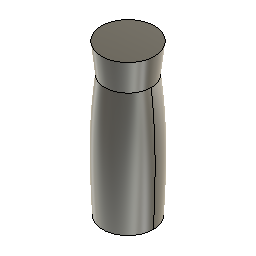
bicycle and bottle_final (Autodesk Fusion 360 archive; units mm, degrees)
design "Bottle"
Autodesk Fusion 360 part; units mm, degrees
sketch "Sketch2" plane through (0, 0, 0) normal (0, 1, 0) x (1, 0, 0)
  line L0 (0, 0) -> (0, -210)
  line L1 (0, -210) -> (36.8, -210)
  line L2 (36.8, -210) -> (32.35, -170)
  line L3 (35.4, 0) -> (0, 0)
  line L4 (32.35, -170) -> (0, -170) construction
  spline S0 degree 5 poles (32.35, -170) (32.7061, -167.196) (33.3914, -161.5338) (34.3388, -152.8777) (35.4383, -141.0057) (36.5224, -125.5792) (37.294, -109.5216) (37.7338, -92.7939) (37.8425, -75.3974) (37.643, -57.3785) (37.1635, -38.7939) (36.5763, -23.5151) (36.029, -11.8401) (35.6175, -3.9624) (35.4, 0) knots 0 0 0 0 0 0 0.1 0.2 0.3 0.4 0.5 0.6 0.7 0.8 0.9 1 1 1 1 1 1
  point P0 (37.5, -100)
  dimension "d13" = 210
  dimension "d14" = 35.4
  dimension "d15" = 36.8
  dimension "d16" = 32.35
  dimension "d18" = 170
  dimension "d20" = 37.5
  dimension "d21" = 100
  constraint coincident L0.start L3.end
  constraint vertical L0
  constraint perpendicular L0 L1
  constraint perpendicular L0 L3
  constraint coincident L0 L4.end
  constraint perpendicular L0 L4
  measures "d13" distance of L0.start L0.end
  measures "d14" distance of L3.start L0.start
  measures "d15" distance of L0.end L1.end
  measures "d16" distance of L0 L2.end
  measures "d18" distance of L3 L4
  measures "d20" distance of L0 P0
  measures "d21" distance of L3 P0
revolve "Revolve1" add sketch "Sketch2" angle 360 about axis through (0, 0, 0) along (0, 0, 1)
equation "overallHeight = 210 mm"
equation "bottomDiameter = ( 70.8 / 2 ) * 1 mm"
equation "bottleCapTop = ( 73.6 / 2 ) * 1 mm"
equation "bottleCapBottom = ( 64.7 / 2 ) * 1 mm"
equation "midDiameter = ( 75 / 2 ) * 1 mm"
equation "bottleBodyHeight = 170 mm" comment "Height to Cap"
equation "midHeight = 100 mm"
equation "d13 = overallHeight"
equation "d14 = bottomDiameter"
equation "d15 = bottleCapTop"
equation "d16 = bottleCapBottom"
equation "d18 = bottleBodyHeight"
equation "d20 = midDiameter"
equation "d21 = midHeight"
